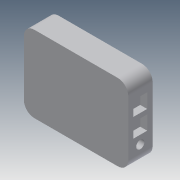
# Autodesk Inventor part: radio
Saved by Autodesk Inventor 2014 (Build 180170000, 170)
## iProperties
Created: 2016-01-12
Part Number: radio
Material: Generic
Document SubType Name: Modeling
Designer: Paul
Density: 1 g/cm^3
Appearance: Default
Author: Paul
Autodesk Inventor part; units mm, degrees
ref_plane "YZ Plane" through (0, 0, 0) normal (1, 0, 0) x (0, 1, 0)
ref_plane "XZ Plane" through (0, 0, 0) normal (0, 1, 0) x (-1, 0, 0)
ref_plane "XY Plane" through (0, 0, 0) normal (0, 0, 1) x (1, 0, 0)
sketch "Sketch1" plane through (0, 0, 0) normal (0, 0, 1) x (1, 0, 0)
  line L0 (9.525, 0) -> (85.725, 0)
  line L1 (95.25, 9.525) -> (95.25, 60.325)
  line L2 (85.725, 69.85) -> (9.525, 69.85)
  line L3 (0, 60.325) -> (0, 9.525)
  arc A0 (9.525, 69.85) -> (0, 60.325) centre (9.525, 60.325) ccw
  arc A1 (95.25, 60.325) -> (85.725, 69.85) centre (85.725, 60.325) ccw
  arc A2 (85.725, 0) -> (95.25, 9.525) centre (85.725, 9.525) ccw
  arc A3 (0, 9.525) -> (9.525, 0) centre (9.525, 9.525) ccw
  point P0 (0, 0)
  point P1 (95.25, 69.85)
  point P2 (95.25, 0)
  point P3 (0, 69.85)
  dimension "d0" = 95.25
  dimension "d1" = 69.85
  dimension "d2" = 9.525
  constraints: 8 end point, 8 point on circle, 8 point on line, 8 tangent, 4 centre point, 3 equal radius, 2 parallel, 1 horizontal, 1 perpendicular
  measures "d0" distance of point (0, 69.85) point (95.25, 69.85)
  measures "d1" distance of point (95.25, 69.85) point (95.25, 0)
  measures "d2" radius of A0
extrude "Extrusion1" add sketch "Sketch1" along normal blind 22.225
sketch "Sketch2" plane through (95.25, 9.525, 0) normal (1, 0, 0) x (0, 0, -1)
  line L0 (-17.5741, 45.1512) -> (-4.9588, 45.1512)
  line L1 (-4.9588, 45.1512) -> (-4.9588, 31.9625)
  line L2 (-4.9588, 31.9625) -> (-17.5741, 31.9625)
  line L3 (-17.5741, 31.9625) -> (-17.5741, 45.1512)
  line L4 (-17.5741, 27.6619) -> (-4.9588, 27.6619)
  line L5 (-4.9588, 27.6619) -> (-4.9588, 14.7599)
  line L6 (-4.9588, 14.7599) -> (-17.5741, 14.7599)
  line L7 (-17.5741, 14.7599) -> (-17.5741, 27.6619)
  circle A0 centre (-11.2665, 7.0188) radius 3.7382
  point P0 (0, -9.525)
  constraints: 16 end point, 4 parallel, 2 horizontal, 2 perpendicular, 1 centre point
extrude "Extrusion2" cut sketch "Sketch2" against normal blind 6.35
sketch "Sketch3" plane through (0, 0, 0) normal (0, 0, -1) x (-1, 0, 0)
  arc A0 (-85.725, 69.85) -> (-95.25, 60.325) centre (-85.725, 60.325) ccw projected
  arc A1 (-95.25, 9.525) -> (-85.725, 0) centre (-85.725, 9.525) ccw projected
  arc A2 (-9.525, 0) -> (0, 9.525) centre (-9.525, 9.525) ccw projected
  arc A3 (0, 60.325) -> (-9.525, 69.85) centre (-9.525, 60.325) ccw projected
  circle A4 centre (-85.725, 60.325) radius 4.7625
  circle A5 centre (-9.525, 60.325) radius 4.7625
  circle A6 centre (-85.725, 9.525) radius 4.7625
  circle A7 centre (-9.525, 9.525) radius 4.7625
  point P0 (0, 0)
  dimension "d7" = 9.525
  dimension "d8" = 9.525
  dimension "d9" = 9.525
  dimension "d10" = 9.525
  constraints: 4 centre point, 4 coincident
  measures "d7" diameter of A4
  measures "d8" diameter of A5
  measures "d9" diameter of A6
  measures "d10" diameter of A7
extrude "Extrusion3" add sketch "Sketch3" along normal blind 3.175
body "Solid1"
